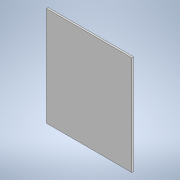
# Autodesk Inventor part: rear_case
Saved by Autodesk Inventor 2022.1 (Build 261234020, 234B)
## iProperties
Created: 2022-02-07
Part Number: rear_case
Material: Generic
Document SubType Name: Modeling
Designer: kee
Density: 1 g/cm^3
Appearance: Default
Mass: 355.86 g
Surface Area: 1476.95 cm^2
Volume: 355.86 cm^3
Author: kee
Autodesk Inventor part; units mm, degrees
ref_plane "YZ Plane" through (0, 0, 0) normal (1, 0, 0) x (0, 1, 0)
ref_plane "XZ Plane" through (0, 0, 0) normal (0, 1, 0) x (-1, 0, 0)
ref_plane "XY Plane" through (0, 0, 0) normal (0, 0, 1) x (1, 0, 0)
sketch "Sketch3" plane through (0, 0, 0) normal (0, 0, 1) x (1, 0, 0)
  line L0 (133.8867, 146.9235) -> (-113.1932, 146.9235)
  line L1 (-113.1932, 146.9235) -> (-113.1932, -141.1294)
  line L2 (-113.1932, -141.1294) -> (133.8867, -141.1294)
  line L3 (133.8867, -141.1294) -> (133.8867, 146.9235)
  point P0 (0, 0)
  constraints: 8 end point, 2 parallel, 1 horizontal, 1 perpendicular
extrude "Extrusion3" add sketch "Sketch3" along normal blind 5
body "Solid2"
